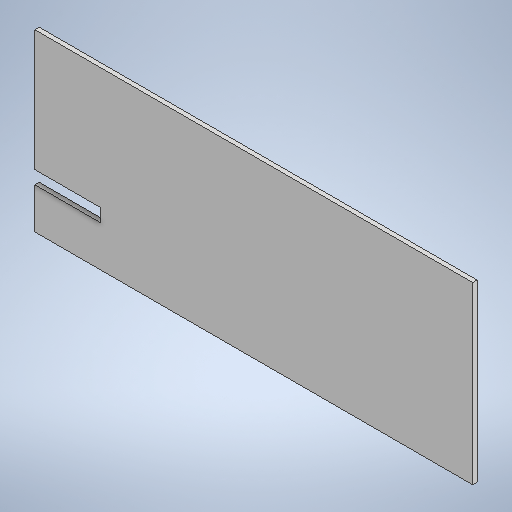
# Autodesk Inventor part: base_01[1]
Saved by Autodesk Inventor 2025.2 (Build 292293000, 293)
## iProperties
Created: 2025-02-06
Part Number: base_01[1]
Material: Generic
Document SubType Name: Modeling
Designer: mpava
Density: 1 g/cm^3
Appearance: Default
Author: mpava
Autodesk Inventor part; units mm, degrees
ref_plane "YZ Plane" through (0, 0, 0) normal (1, 0, 0) x (0, 1, 0)
ref_plane "XZ Plane" through (0, 0, 0) normal (0, 1, 0) x (-1, 0, 0)
ref_plane "XY Plane" through (0, 0, 0) normal (0, 0, 1) x (1, 0, 0)
sketch "Sketch1" plane through (0, 0, 0) normal (0, 0, 1) x (1, 0, 0)
  line L0 (-150, 60) -> (150, 60)
  line L1 (150, 60) -> (150, -60)
  line L2 (150, -60) -> (-150, -60)
  line L3 (-150, -60) -> (-150, 60)
  line L4 (-150, 60) -> (150, -60) construction
  line L5 (150, 60) -> (-150, -60) construction
  point P0 (0, 0)
  dimension "d0" = 300
  dimension "d1" = 120
  constraints: 12 end point, 2 midpoint, 2 parallel, 1 horizontal, 1 perpendicular
  measures "d0" distance of L1.end L2.end
  measures "d1" distance of L0.end L1.end
extrude "Extrusion1" add sketch "Sketch1" along normal blind 3
sketch "Sketch2" plane through (0, 0, 3) normal (0, 0, 1) x (1, 0, 0)
  line L0 (-150, -32) -> (-105, -32)
  line L1 (-105, -32) -> (-105, -23)
  line L2 (-105, -23) -> (-150, -23)
  line L3 (-150, -23) -> (-150, -32)
  point P0 (0, 0)
  dimension "d4" = 45
  dimension "d5" = 9
  constraints: 8 end point, 2 parallel, 1 horizontal, 1 perpendicular
  measures "d4" distance of L2.end L1.end
  measures "d5" distance of L1.end L0.end
extrude "Extrusion2" cut sketch "Sketch2" against normal up to surface (3 mm away)
body "Solid1"
